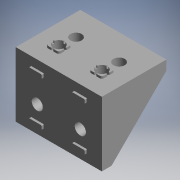
# Autodesk Inventor part: HBLFSD5-SECh5
Saved by Autodesk Inventor 2017.3 (Build 213256000, 256)
## iProperties
Part Number: HBLFSD5-SECh5
Material: Generic
Catalog Web Link: www.cadenas.de
Description: HBLFSN5, HBLFSNB5, HBLFSNM5, HBLFSNK5, HBLFSSW5, HBLFSSWB5, HBLFSDW5-Thin Reversal Brackets for Slot Width 6 Frames - For 20, 40mm Sections
Vendor: MISUMI
Document SubType Name: Modeling
Designer: partserver
Manufacturer: MISUMI
Mass: 10.6442 g
Surface Area: 68.7333 cm^2
Volume: 10.6442 cm^3
Density: 1 g/cm^3
Appearance: PSOLRGB-192-192-192
Category: PARTsolutions
Company: MISUMI
Title: HBLFSD5-SEC
Author: Cadenas PARTsolutions
Comments: Thin Reversal Brackets for Slot Width 6 Frames - For 20, 40mm Sections
PSOL_IDENT_0: {$CADENAS_DATA\23d-libs\misumi\metric\38_al_extrusions_blackets\5\hblfsn5.prj},236 {VTYP=3D},{NB=HBL
PSOL_IDENT_1: FSD5-SECh5},{LINA=HBLFSD5-SEC},{NN=HBLFSN5, HBLFSNB5, HBLFSNM5, HBLFSNK5, HBLFSSW5, HBLFSSWB5, HBLFS
PSOL_IDENT_2: DW5},{DATE=16.10.2018 09:36:58},{GEOMDATE=16.10.2018 09:22:00},{VERSION=},{LINEID=270},{WBVAR=ALT1,A
PSOL_IDENT_3: LT2},{WBNUMERIC=}  {NB=HBLFSD5-SECh5},{LINA=HBLFSD5-SEC},{KT=5},{PN=HBLFSD5-SEC},{TP=HBLFSD5},{NOH=2
PSOL_IDENT_4: },{NOHV=2},{MAT=JIS-ADC12},{ST=-},{TYPE=HBLFSD5},{FEAT=Thin Reversal Bracket},{ALT1=},{ALT2=-SEC},{M
PSOL_IDENT_5: ASS=25},{AB=CBM5-10},{NOB=4},{AN=HNTT5-5},{NON=4},{AL=1470},{W=40},{H=30},{DP=30},{T=4.5},{HDIS=0},{
PSOL_IDENT_6: DPOS=12},{HH1=18},{BOLTX=0.0},{HV1=0},{BOLTY=0.0},{DIA=5.2},{ALT1OPT='','w/o C (Mounting Holes for C
PSOL_IDENT_7: over)','-C','with C (Mounting Holes for Cover)'},{ALT2OPT= '' , 'w/o Set of Applicable Bolt and Nut'
PSOL_IDENT_8: , '-SET' , 'with SET (Set of Applicable Bolt and Nut)' , '-SST' , 'with SST (Stainless Steel Set of
PSOL_IDENT_9: Applicable Bolt and Nut)' , '-SEU' , 'with SEU (Pre-Assembly Fitting Spring Nuts Set of Applicable
PSOL_IDENT_10: Bolt and Nut)' , '-SSU' , 'with SSU (Pre-Assembly Fitting Spring Nuts Stainless Set of Applicable Bo
PSOL_IDENT_11: lt and Nut)'  , '-SEP' , 'with SEP (Post-Assembly Fitting Spring Nuts Set of Applicable Bolt and Nut
PSOL_IDENT_12: )' , '-SSP' , 'with SSP (Post-Assembly Fitting Spring Nuts Stainless Set of Applicable Bolt and Nut)'
PSOL_IDENT_13: , '-SEC' , 'with SEC (Washer Assembled Set of Applicable Bolt and Nut)' },{R=1},{R1=0.3},{APOSV=0}
PSOL_IDENT_14: ,{VER=3},{PR=5},{TT=1.0},{T1=0}
NB: HBLFSD5-SECh5
NN: HBLFSN5, HBLFSNB5, HBLFSNM5, HBLFSNK5, HBLFSSW5, HBLFSSWB5, HBLFSDW5
NT: Thin Reversal Brackets for Slot Width 6 Frames - For 20, 40mm Sections
NBSYN: $PN.h5
LINA: HBLFSD5-SEC
CATALOG: Misumi
PN: HBLFSD5-SEC
TP: HBLFSD5
MAT: JIS-ADC12
ST: -
FEAT: Thin Reversal Bracket
ALT1: w/o C (Mounting Holes for Cover)
ALT2: with SEC (Washer Assembled Set of Applicable Bolt and Nut)
MASS: 25
AB: CBM5-10
NOB: 4
AN: HNTT5-5
NON: 4
AL: 1470
BOLTX: 0
BOLTY: 0
SUPPLIER: MISUMI
ARTICLENO: HBLFSD5-SECh5
BOMINFO: HBLFSD5-SEC
CREATOR: CADENAS GmbH
Autodesk Inventor part; units mm, degrees
ref_plane "YZ Plane" through (0, 0, 0) normal (1, 0, 0) x (0, 1, 0)
ref_plane "XZ Plane" through (0, 0, 0) normal (0, 1, 0) x (-1, 0, 0)
ref_plane "XY Plane" through (0, 0, 0) normal (0, 0, 1) x (1, 0, 0)
sketch "Sketch_15" plane through (0, 0, 0) normal (1, 0, 0) x (0, 1, 0)
  line L0 (4.0858, 30) -> (0, 30)
  line L1 (0, 30) -> (0, 0)
  line L2 (0, 0) -> (30, 0)
  line L3 (30, 0) -> (30, 4.0858)
  arc A0 (30, 4.0858) -> (29.7071, 4.7929) centre (29, 4.0858) ccw
  line L4 (29.7071, 4.7929) -> (4.7929, 29.7071)
  arc A1 (4.7929, 29.7071) -> (4.0858, 30) centre (4.0858, 29) ccw
  constraints: 10 end point, 4 point on circle, 2 centre point
extrude "Extrusion1" add sketch "Sketch_15" along normal mid plane 40
sketch "Sketch_16" plane through (0, 0, 0) normal (1, 0, 0) x (0, 1, 0)
  line L0 (34.5, 34.5) -> (2.9278, 34.5)
  line L1 (2.9278, 34.5) -> (4.5, 4.5)
  line L2 (4.5, 4.5) -> (34.5, 4.5)
  line L3 (34.5, 4.5) -> (34.5, 34.5)
  constraints: 8 end point
extrude "Extrusion2" cut sketch "Sketch_16" along normal mid plane 35
sketch "Sketch_34" plane through (0, 4.5, 0) normal (0, 1, 0) x (1, 0, 0)
  line L0 (4.5791, -10.5) -> (5.5313, -18.5299)
  arc A0 (5.5313, -18.5299) -> (14.4687, -18.5299) centre (10, -18) ccw
  line L1 (14.4687, -18.5299) -> (15.4209, -10.5)
  line L2 (15.4209, -10.5) -> (4.5791, -10.5)
  constraints: 6 end point, 2 point on circle, 1 centre point
extrude "Extrusion3" add sketch "Sketch_34" against normal blind 2.25
sketch "Sketch_35" plane through (0, 4.5, 0) normal (0, 1, 0) x (1, 0, 0)
  line L0 (-15.4209, -10.5) -> (-14.4687, -18.5299)
  arc A0 (-14.4687, -18.5299) -> (-5.5313, -18.5299) centre (-10, -18) ccw
  line L1 (-5.5313, -18.5299) -> (-4.5791, -10.5)
  line L2 (-4.5791, -10.5) -> (-15.4209, -10.5)
  constraints: 6 end point, 2 point on circle, 1 centre point
extrude "Extrusion4" add sketch "Sketch_35" against normal blind 2.25
sketch "Sketch5" plane through (-20, 0, 0) normal (0, -1, 0) x (1, 0, 0)
  point P0 (30, 18)
hole "Hole1" at (10, 0, 18) direction (0, 1, 0) diameter 5.2 depth 4.5
sketch "Sketch6" plane through (-20, 0, 0) normal (0, -1, 0) x (1, 0, 0)
  point P0 (10, 18)
hole "Hole2" at (-10, 0, 18) direction (0, 1, 0) diameter 5.2 depth 4.5
sketch "Sketch_32" plane through (0, 0, 0) normal (0, 0, 1) x (1, 0, 0)
  circle A0 centre (-10, 10) radius 2.6
  constraints: 1 centre point
extrude "Extrusion5" cut sketch "Sketch_32" along normal mid plane 35
pattern_linear "Rectangular Pattern1" count 2 spacing 20 along (1, 0, 0) count 2 spacing 8 along (0, 1, 0) of "Extrusion5"
sketch "Sketch_1" plane through (0, 0, 0) normal (0, 1, 0) x (-1, 0, 0)
  line L0 (20, 30) -> (-20, 30)
  line L1 (-20, 30) -> (-20, 0)
  line L2 (-20, 0) -> (20, 0)
  line L3 (20, 0) -> (20, 30)
  constraints: 8 end point
extrude "Extrusion6" add sketch "Sketch_1" against normal blind 1
sketch "Sketch_38" plane through (0, 0, 0) normal (0, 1, 0) x (-1, 0, 0)
  line L0 (20, 30) -> (-20, 30)
  line L1 (-20, 30) -> (-20, 0)
  line L2 (-20, 0) -> (20, 0)
  line L3 (20, 0) -> (20, 30)
  line L4 (-7, 24.8) -> (-7, 26.2)
  arc A0 (-7, 26.2) -> (-7.3, 26.5) centre (-7.3, 26.2) ccw
  line L5 (-7.3, 26.5) -> (-12.7, 26.5)
  arc A1 (-12.7, 26.5) -> (-13, 26.2) centre (-12.7, 26.2) ccw
  line L6 (-13, 26.2) -> (-13, 24.8)
  arc A2 (-13, 24.8) -> (-12.7, 24.5) centre (-12.7, 24.8) ccw
  line L7 (-12.7, 24.5) -> (-7.3, 24.5)
  arc A3 (-7.3, 24.5) -> (-7, 24.8) centre (-7.3, 24.8) ccw
  line L8 (-7, 4.3) -> (-7, 5.7)
  arc A4 (-7, 5.7) -> (-7.3, 6) centre (-7.3, 5.7) ccw
  line L9 (-7.3, 6) -> (-12.7, 6)
  arc A5 (-12.7, 6) -> (-13, 5.7) centre (-12.7, 5.7) ccw
  line L10 (-13, 5.7) -> (-13, 4.3)
  arc A6 (-13, 4.3) -> (-12.7, 4) centre (-12.7, 4.3) ccw
  line L11 (-12.7, 4) -> (-7.3, 4)
  arc A7 (-7.3, 4) -> (-7, 4.3) centre (-7.3, 4.3) ccw
  line L12 (13, 24.8) -> (13, 26.2)
  arc A8 (13, 26.2) -> (12.7, 26.5) centre (12.7, 26.2) ccw
  line L13 (12.7, 26.5) -> (7.3, 26.5)
  arc A9 (7.3, 26.5) -> (7, 26.2) centre (7.3, 26.2) ccw
  line L14 (7, 26.2) -> (7, 24.8)
  arc A10 (7, 24.8) -> (7.3, 24.5) centre (7.3, 24.8) ccw
  line L15 (7.3, 24.5) -> (12.7, 24.5)
  arc A11 (12.7, 24.5) -> (13, 24.8) centre (12.7, 24.8) ccw
  line L16 (13, 4.3) -> (13, 5.7)
  arc A12 (13, 5.7) -> (12.7, 6) centre (12.7, 5.7) ccw
  line L17 (12.7, 6) -> (7.3, 6)
  arc A13 (7.3, 6) -> (7, 5.7) centre (7.3, 5.7) ccw
  line L18 (7, 5.7) -> (7, 4.3)
  arc A14 (7, 4.3) -> (7.3, 4) centre (7.3, 4.3) ccw
  line L19 (7.3, 4) -> (12.7, 4)
  arc A15 (12.7, 4) -> (13, 4.3) centre (12.7, 4.3) ccw
  constraints: 40 end point, 32 point on circle, 16 centre point
extrude "Extrusion7" cut sketch "Sketch_38" against normal blind 1
sketch "Sketch_10" plane through (0, 0, 0) normal (0, 0, 1) x (1, 0, 0)
  line L0 (-20, 30) -> (-20, 0)
  line L1 (-20, 0) -> (20, 0)
  line L2 (20, 0) -> (20, 30)
  line L3 (20, 30) -> (-20, 30)
  constraints: 8 end point
extrude "Extrusion8" add sketch "Sketch_10" against normal blind 1
sketch "Sketch_39" plane through (0, 0, 0) normal (0, 0, 1) x (1, 0, 0)
  line L0 (-20, 30) -> (-20, 0)
  line L1 (-20, 0) -> (20, 0)
  line L2 (20, 0) -> (20, 30)
  line L3 (20, 30) -> (-20, 30)
  arc A0 (12.5515, 10.5) -> (10.5, 12.5515) centre (10, 10) ccw
  line L4 (12.5515, 10.5) -> (13, 10.5)
  line L5 (13, 10.5) -> (13, 12)
  arc A1 (13, 12) -> (12, 13) centre (12, 12) ccw
  line L6 (12, 13) -> (10.5, 13)
  line L7 (10.5, 13) -> (10.5, 12.5515)
  line L8 (10.5, 7.4485) -> (10.5, 7)
  line L9 (10.5, 7) -> (12, 7)
  arc A2 (12, 7) -> (13, 8) centre (12, 8) ccw
  line L10 (13, 8) -> (13, 9.5)
  line L11 (13, 9.5) -> (12.5515, 9.5)
  arc A3 (10.5, 7.4485) -> (12.5515, 9.5) centre (10, 10) ccw
  line L12 (7, 12) -> (7, 10.5)
  line L13 (7, 10.5) -> (7.4485, 10.5)
  arc A4 (9.5, 12.5515) -> (7.4485, 10.5) centre (10, 10) ccw
  line L14 (9.5, 12.5515) -> (9.5, 13)
  line L15 (9.5, 13) -> (8, 13)
  arc A5 (8, 13) -> (7, 12) centre (8, 12) ccw
  line L16 (7, 9.5) -> (7, 8)
  arc A6 (7, 8) -> (8, 7) centre (8, 8) ccw
  line L17 (8, 7) -> (9.5, 7)
  line L18 (9.5, 7) -> (9.5, 7.4485)
  arc A7 (7.4485, 9.5) -> (9.5, 7.4485) centre (10, 10) ccw
  line L19 (7.4485, 9.5) -> (7, 9.5)
  arc A8 (-7.4485, 10.5) -> (-9.5, 12.5515) centre (-10, 10) ccw
  line L20 (-7.4485, 10.5) -> (-7, 10.5)
  line L21 (-7, 10.5) -> (-7, 12)
  arc A9 (-7, 12) -> (-8, 13) centre (-8, 12) ccw
  line L22 (-8, 13) -> (-9.5, 13)
  line L23 (-9.5, 13) -> (-9.5, 12.5515)
  line L24 (-9.5, 7.4485) -> (-9.5, 7)
  line L25 (-9.5, 7) -> (-8, 7)
  arc A10 (-8, 7) -> (-7, 8) centre (-8, 8) ccw
  line L26 (-7, 8) -> (-7, 9.5)
  line L27 (-7, 9.5) -> (-7.4485, 9.5)
  arc A11 (-9.5, 7.4485) -> (-7.4485, 9.5) centre (-10, 10) ccw
  line L28 (-13, 12) -> (-13, 10.5)
  line L29 (-13, 10.5) -> (-12.5515, 10.5)
  arc A12 (-10.5, 12.5515) -> (-12.5515, 10.5) centre (-10, 10) ccw
  line L30 (-10.5, 12.5515) -> (-10.5, 13)
  line L31 (-10.5, 13) -> (-12, 13)
  arc A13 (-12, 13) -> (-13, 12) centre (-12, 12) ccw
  line L32 (-13, 9.5) -> (-13, 8)
  arc A14 (-13, 8) -> (-12, 7) centre (-12, 8) ccw
  line L33 (-12, 7) -> (-10.5, 7)
  line L34 (-10.5, 7) -> (-10.5, 7.4485)
  arc A15 (-12.5515, 9.5) -> (-10.5, 7.4485) centre (-10, 10) ccw
  line L35 (-12.5515, 9.5) -> (-13, 9.5)
  constraints: 72 end point, 32 point on circle, 16 centre point
extrude "Extrusion9" cut sketch "Sketch_39" against normal blind 1
ref_plane "bolt_10_11_base_1_XY" through (-10, 4.5, 18) normal (0, 1, 0) x (1, 0, 0)
ref_plane "bolt_10_11_base_1_YZ" through (-10, 4.5, 18) normal (1, 0, 0) x (0, 0, -1)
ref_plane "bolt_10_11_base_1_ZX" through (-10, 4.5, 18) normal (0, 0, -1) x (0, 1, 0)
ref_plane "bolt_10_11_base_2_XY" through (10, 4.5, 18) normal (0, 1, 0) x (1, 0, 0)
ref_plane "bolt_10_11_base_2_YZ" through (10, 4.5, 18) normal (1, 0, 0) x (0, 0, -1)
ref_plane "bolt_10_11_base_2_ZX" through (10, 4.5, 18) normal (0, 0, -1) x (0, 1, 0)
ref_plane "bracket_to_bolt_XY" through (1, 0, 0) normal (0, 0, 1) x (1, 0, 0)
ref_plane "bracket_to_bolt_YZ" through (1, 0, 0) normal (1, 0, 0) x (0, 1, 0)
ref_plane "bracket_to_bolt_ZX" through (1, 0, 0) normal (0, 1, 0) x (0, 0, 1)
ref_plane "bracket_to_dummy_XY" through (0, 0, 0) normal (0, 1, 0) x (1, 0, 0)
ref_plane "bracket_to_dummy_YZ" through (0, 0, 0) normal (1, 0, 0) x (0, 0, -1)
ref_plane "bracket_to_dummy_ZX" through (0, 0, 0) normal (0, 0, -1) x (0, 1, 0)
ref_plane "nut_10_11_base_1_XY" through (-10, -2, 18) normal (0, 1, 0) x (1, 0, 0)
ref_plane "nut_10_11_base_1_YZ" through (-10, -2, 18) normal (1, 0, 0) x (0, 0, -1)
ref_plane "nut_10_11_base_1_ZX" through (-10, -2, 18) normal (0, 0, -1) x (0, 1, 0)
ref_plane "nut_10_11_base_2_XY" through (10, -2, 18) normal (0, 1, 0) x (1, 0, 0)
ref_plane "nut_10_11_base_2_YZ" through (10, -2, 18) normal (1, 0, 0) x (0, 0, -1)
ref_plane "nut_10_11_base_2_ZX" through (10, -2, 18) normal (0, 0, -1) x (0, 1, 0)
ref_plane "to_bolt_row_10_11_1_XY" through (-10, 18, 4.5) normal (0, 0, 1) x (1, 0, 0)
ref_plane "to_bolt_row_10_11_1_YZ" through (-10, 18, 4.5) normal (1, 0, 0) x (0, 1, 0)
ref_plane "to_bolt_row_10_11_1_ZX" through (-10, 18, 4.5) normal (0, 1, 0) x (0, 0, 1)
ref_plane "to_bolt_row_10_11_2_XY" through (10, 18, 4.5) normal (0, 0, 1) x (1, 0, 0)
ref_plane "to_bolt_row_10_11_2_YZ" through (10, 18, 4.5) normal (1, 0, 0) x (0, 1, 0)
ref_plane "to_bolt_row_10_11_2_ZX" through (10, 18, 4.5) normal (0, 1, 0) x (0, 0, 1)
ref_plane "to_nut_row_10_11_1_XY" through (-10, 18, -2) normal (0, 0, 1) x (1, 0, 0)
ref_plane "to_nut_row_10_11_1_YZ" through (-10, 18, -2) normal (1, 0, 0) x (0, 1, 0)
ref_plane "to_nut_row_10_11_1_ZX" through (-10, 18, -2) normal (0, 1, 0) x (0, 0, 1)
ref_plane "to_nut_row_10_11_2_XY" through (10, 18, -2) normal (0, 0, 1) x (1, 0, 0)
ref_plane "to_nut_row_10_11_2_YZ" through (10, 18, -2) normal (1, 0, 0) x (0, 1, 0)
ref_plane "to_nut_row_10_11_2_ZX" through (10, 18, -2) normal (0, 1, 0) x (0, 0, 1)
body "Solid1"
